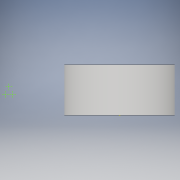
# Autodesk Inventor part: working VBA
Saved by Autodesk Inventor 2018 (Build 220112000, 112)
## iProperties
Created: 2018-09-01
Part Number: working VBA
Material: Generic
Document SubType Name: Modeling
Designer: Nun Maker
Density: 1 g/cm^3
Appearance: Default
Author: Nun Maker
Autodesk Inventor part; units mm, degrees
ref_plane "YZ Plane" through (0, 0, 0) normal (1, 0, 0) x (0, 1, 0)
ref_plane "XZ Plane" through (0, 0, 0) normal (0, 1, 0) x (-1, 0, 0)
ref_plane "XY Plane" through (0, 0, 0) normal (0, 0, 1) x (1, 0, 0)
sketch "Sketch1" plane through (0, 0, 0) normal (0, 0, 1) x (1, 0, 0)
  line L0 (9.497, 0) -> (11.1029, 0)
  line L1 (11.1029, 0) -> (11.1029, 10.0665)
  line L2 (11.1029, 10.0665) -> (9.497, 10.0665)
  line L3 (9.497, 10.0665) -> (9.497, 0)
  line L4 (0, -2.0133) -> (0, 12.0798) projected
  point P0 (0, 0)
  dimension "d0" = 10.0665
  dimension "d1" = 9.497
  dimension "d14" = 14.8028
  constraints: 8 end point, 2 parallel, 1 horizontal, 1 perpendicular
  measures "d0" distance of L0.end L1.end
  measures "d1" distance of L0.start point (0, 0)
revolve "Revolution1" add sketch "Sketch1" angle 360 about axis through (0, -10, 0) along (0, 1, 0)
sketch "Sketch18" plane through (0, 0, 0) normal (0, 0, 1) x (1, 0, 0)
  point P0 (0, 0)
  point P1 (-22.2647, 5.6563)
  point P2 (-21.5147, 4.1563)
  point P3 (-23.0147, 4.1563)
equation "\"d0\" = height"
equation "\"ri\" = 9.5"
equation "\"height\" = 10.06647"
equation "\"l_t\" = 10.7"
equation "\"s_t\" = 0.46188"
equation "\"dr\" = 0.666667"
equation "\"d119\" = 9.2"
equation "\"d133\" = 9.2"
equation "\"d149\" = 9.2"
equation "\"d160\" = 9.2"
equation "\"wt\" = 0.4"
equation "\"d170\" = 0.3"
equation "\"d176\" = 0.3"
equation "\"d180\" = 9.2"
equation "\"d181\" = 0.3"
equation "\"loss\" = 0.003"
body "Solid1"
